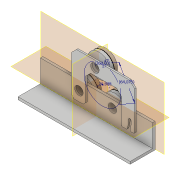
# Autodesk Inventor part: Part1
Saved by Autodesk Inventor 2019 (Build 230136000, 136)
## iProperties
Created: 2019-11-14
Part Number: Part1
Material: Generic
Document SubType Name: Modeling
Designer: Carlos Andres garcia velez
Density: 1 g/cm^3
Appearance: Default
Author: Carlos Andres garcia velez
Autodesk Inventor part; units mm, degrees
sketch "Sketch1" plane through (0, 0, 0) normal (0, 0, 1) x (1, 0, 0)
  circle A0 centre (0, 0) radius 13.4938 construction
  circle A1 centre (0, 36.9937) radius 8.5
  circle A2 centre (0, 36.9937) radius 23.5
  circle A3 centre (-32.0375, -18.4969) radius 23.5
  circle A4 centre (-32.0375, -18.4969) radius 8.5
  circle A5 centre (32.0375, -18.4969) radius 23.5
  circle A6 centre (32.0375, -18.4969) radius 8.5
  dimension "d0" = 26.9875
  dimension "d1" = 17
  dimension "d2" = 47
  dimension "d5" = 360
  dimension "d25" = 64.0751
  constraints: 7 centre point, 4 coincident, 1 tangent, 13 other
  measures "d0" diameter of A0
  measures "d1" diameter of A1
  measures "d2" diameter of A2
  measures "d25" distance of A6.centre A1.centre
extrude "Extrusion1" add sketch "Sketch1" along normal mid plane 14
sketch "Sketch4" plane through (32.0375, -18.4969, 7) normal (0, 0, 1) x (1, 0, 0)
  line L0 (-144.5375, -35) -> (80.4625, -35)
  line L1 (80.4625, -35) -> (80.4625, 15)
  line L2 (80.4625, 15) -> (-144.5375, 15)
  line L3 (-144.5375, 15) -> (-144.5375, -35)
  line L4 (-144.5375, -35) -> (80.4625, 15) construction
  line L5 (80.4625, -35) -> (-144.5375, 15) construction
  line L6 (-32.0375, 101.7888) -> (-32.0375, -57.7981) projected
  circle A0 centre (0, 0) radius 8.5 projected
  circle A1 centre (-64.0751, 0) radius 8.5 projected
  point P0 (-32.0375, 18.4969)
  point P1 (-32.0375, -10)
  dimension "d16" = 50
  dimension "d17" = 225
  dimension "d18" = 0
  dimension "d19" = 15
  constraints: 12 end point, 2 midpoint, 2 parallel, 1 horizontal, 1 perpendicular
  measures "d16" distance of L1.end L0.end
  measures "d17" distance of L1.end L2.end
  measures "d18" distance from line of point (-32.038, -10) L6
  measures "d19" distance from line of A0.centre L2
extrude "Extrusion3" add sketch "Sketch4" along normal blind 5
sketch "Sketch5" plane through (32.0375, -18.4969, 12) normal (0, 0, 1) x (1, 0, 0)
  line L0 (-144.5375, -35) -> (80.4625, -35) projected
  line L1 (-144.5375, 15) -> (-144.5375, -35) projected
  line L2 (80.4625, -35) -> (80.4625, 15) projected
  line L3 (-144.5375, -30) -> (80.4625, -30)
  point P0 (-32.0375, 18.4969)
  dimension "d22" = 5
  constraints: 2 end point, 2 point on line, 1 perpendicular
  measures "d22" distance between parallel lines of L0 L3
extrude "Extrusion4" add sketch "Sketch5" along normal blind 45
sketch "Sketch6" plane through (32.0375, -18.4969, 12) normal (0, 0, 1) x (1, 0, 0)
  circle A0 centre (-32.0375, 18.4969) radius 13.4938 construction
  circle A1 centre (-32.0375, 55.4906) radius 23.5 projected
  circle A2 centre (-32.0375, 55.4906) radius 8.5 projected
  circle A3 centre (-64.0751, 0) radius 8.5 projected
  circle A4 centre (-64.0751, 0) radius 8.5 projected
  line L0 (47.6707, -19.2354) -> (47.6707, 68.9906)
  line L1 (47.6707, 68.9906) -> (-79.0751, 68.9906)
  line L2 (-79.0751, 68.9906) -> (-79.0751, -19.2354)
  circle A5 centre (-64.0751, 0) radius 23.5 projected
  line L3 (-50.5751, -19.2354) -> (21.6707, -19.2354)
  line L4 (21.6707, -19.2354) -> (21.6707, 41.9906)
  line L5 (21.6707, 41.9906) -> (-50.5751, 41.9906)
  line L6 (-50.5751, 41.9906) -> (-50.5751, -19.2354)
  arc A6 (18.0901, 15) -> (-18.0901, 15) centre (0, 0) ccw projected
  arc A7 (-18.0901, 15) -> (18.0901, 15) centre (0, 0) ccw projected
  arc A8 (35, -19.2354) -> (37.509, -10) centre (-7.2886, -2.7883) ccw construction
  arc A9 (37.8316, -19.2354) -> (40.645, 0.1628) centre (-7.2886, -2.7883) ccw
  arc A10 (32.5302, -18.2748) -> (35.355, -0.1628) centre (-7.2886, -2.7883) ccw
  arc A11 (40.645, 0.1628) -> (35.355, -0.1628) centre (38, 0) ccw
  arc A12 (32.5302, -18.2748) -> (32.35, -19.2354) centre (35, -19.2354) ccw
  line L7 (-79.0751, -19.2354) -> (32.35, -19.2354)
  line L8 (37.8316, -19.2354) -> (47.6707, -19.2354)
  dimension "d26" = 5
  dimension "d27" = 13.5
  dimension "d28" = 15
  dimension "d30" = 13.5
  dimension "d32" = 28.5
  dimension "d33" = 26
  constraints: 18 end point, 10 point on circle, 6 centre point, 5 parallel, 3 horizontal, 3 perpendicular, 3 tangent, 1 coincident, 1 point on line, 2 other
  measures "d26" distance edge to line of A3 L6
  measures "d27" distance from line of A2.centre L5
  measures "d28" distance from line of L2 A3.centre
  measures "d30" distance from line of L1 A2.centre
  measures "d32" distance between parallel lines of L2 L6
  measures "d33" distance between parallel lines of L0 L4
extrude "Extrusion5" add sketch "Sketch6" along normal blind 3.175 separate body contours A1 L5 L6 L1 | A1 L1 L0 L8 A9 A11 A10 A12 L7 L4 A7 L5 | A1 L6 A5 L2 L1 | L6 L7 A5 L2 | A7 L4 | A5 L7 L2
chamfer "Chamfer1" distance 10 angle 45 1 edges at (-18.5375, 23.4938, 13.5875)
chamfer "Chamfer2" distance 10 angle 45 3 edges at (-47.0375, 50.4937, 13.5875) (79.7082, 50.4938, 13.5875) (53.7082, 23.4938, 13.5875)
fillet "Fillet1" radius 2 4 edges at (53.7082, -37.7323, 13.5875) (64.3875, -37.7323, 13.5875) (79.7082, -37.7323, 13.5875) (69.8691, -37.7323, 13.5875)
chamfer "Chamfer3" distance 5 angle 45 2 edges at (-47.0375, -37.7323, 13.5875) (-18.5375, -37.7323, 13.5875)
body "Solid1"
body "Solid2"
